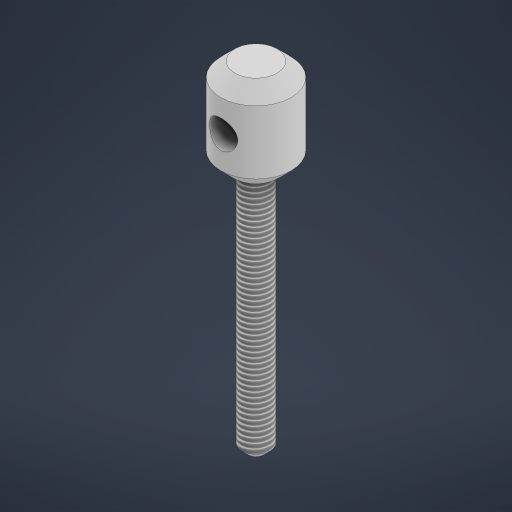
# Autodesk Inventor part: Część29
Saved by Autodesk Inventor 2023 (Build 270158000, 158)
## iProperties
Created: 2023-05-09
Part Number: Część29
Material: Ogólny
Document SubType Name: Modeling
Designer: Adam
Density: 1 g/cm^3
Appearance: Domyślna
Author: Adam
Autodesk Inventor part; units mm, degrees
ref_plane "YZ Plane" through (0, 0, 0) normal (1, 0, 0) x (0, 1, 0)
ref_plane "XZ Plane" through (0, 0, 0) normal (0, 1, 0) x (-1, 0, 0)
ref_plane "XY Plane" through (0, 0, 0) normal (0, 0, 1) x (1, 0, 0)
sketch "Szkic1" plane through (0, 0, 0) normal (1, 0, 0) x (0, 1, 0)
  line L0 (0, 0) -> (0, -2)
  line L1 (0, -2) -> (35, -2)
  line L2 (35, -2) -> (35, -5)
  line L3 (35, -5) -> (48, -5)
  line L4 (48, -5) -> (48, 0)
  line L5 (48, 0) -> (0, 0)
  dimension "d0" = 35
  constraints: 12 end point, 4 perpendicular, 1 parallel, 1 vertical
  measures "d0" distance of L0.end L1.end
revolve "Obrót1" add sketch "Szkic1" angle 360 about axis through (0, 48, 0) along (0, -1, 0)
chamfer "Faza1" distance 2 angle 45 2 edges at (0, 48, 5) (0, 35, 5) measured on face at (-0.4023, 39.3333, -4.9838)
chamfer "Faza2" distance 1 angle 45 1 edges at (0, 0, 2) measured on face at (1.2634, 0, -0.0679)
thread "Gwint1" size "M4x0.7" class "6g" standard "ANSI Metric M Profile" full length
sketch "Szkic2" plane through (0, 0, 0) normal (0, 0, 1) x (1, 0, 0)
  point P0 (0, 0)
  point P1 (0, 41.5)
hole "Otwór1" at (0, 41.5, 0) direction (0, 0, -1) diameter 4 end through all both
